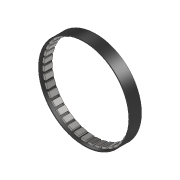
# Autodesk Inventor part: rotor
Saved by Autodesk Inventor 2020 (Build 240168000, 168)
## iProperties
Created: 2020-05-19
Part Number: rotor
Material: Generic
Document SubType Name: Modeling
Designer: Kostic
Density: 1 g/cm^3
Appearance: Glossy - Black
Author: Kostic
Autodesk Inventor part; units mm, degrees
ref_plane "YZ Plane" through (0, 0, 0) normal (1, 0, 0) x (0, 1, 0)
ref_plane "XZ Plane" through (0, 0, 0) normal (0, 1, 0) x (-1, 0, 0)
ref_plane "XY Plane" through (0, 0, 0) normal (0, 0, 1) x (1, 0, 0)
sketch "Sketch1" plane through (0, 0, 0) normal (0, 0, 1) x (1, 0, 0)
  circle A0 centre (0, 0) radius 45.9
  circle A1 centre (0, 0) radius 44.5
  dimension "d0" = 91.8
  dimension "d1" = 89
  constraints: 2 centre point, 2 coincident
  measures "d0" diameter of A0
  measures "d1" diameter of A1
extrude "Extrusion1" add sketch "Sketch1" along normal blind 1
sketch "Sketch2" plane through (0, 0, 1) normal (0, 0, 1) x (1, 0, 0)
  circle A0 centre (0, 0) radius 45.9
  circle A1 centre (0, 0) radius 44.9
  dimension "d4" = 89.8
  dimension "d5" = 91.8
  constraints: 2 centre point, 2 coincident
  measures "d4" diameter of A1
  measures "d5" diameter of A0
extrude "Extrusion2" add sketch "Sketch2" along normal blind 8
sketch "Sketch5" plane through (0, 0, 1) normal (0, 0, 1) x (1, 0, 0)
  line L0 (-2.5, 42.8303) -> (2.5, 42.8303)
  line L1 (2.5, 42.8303) -> (2.5, 44.8303)
  line L2 (2.5, 44.8303) -> (-2.5, 44.8303)
  line L3 (-2.5, 44.8303) -> (-2.5, 42.8303)
  circle A0 centre (0, 0) radius 44.9 projected
  dimension "d8" = 5
  dimension "d9" = 2
  dimension "d10" = 2.5
  constraints: 8 end point, 2 parallel, 1 horizontal, 1 perpendicular, 2 other
  measures "d8" distance of L2.end L1.end
  measures "d9" distance of L1.end L0.end
  measures "d10" distance from line of point (0, 0) L3
extrude "Extrusion3" add sketch "Sketch5" along normal blind 8 contours L3 L2 L1 L0
pattern_circular "Circular Pattern1" count 39 over 360 about axis through (0, 0, 1) along (0, 0, 1) of "Extrusion3"
sketch "Sketch6" plane through (0, 0, 9) normal (0, 0, 1) x (1, 0, 0)
  circle A0 centre (0, 0) radius 45.9
  circle A1 centre (0, 0) radius 44.9
  circle A2 centre (0, 0) radius 45.9 projected
  dimension "d18" = 89.8
  constraints: 2 centre point, 2 coincident, 1 concentric
  measures "d18" diameter of A1
extrude "Extrusion4" add sketch "Sketch6" along normal blind 3
equation "\"d10\" = 0.5 * d8"
body "Solid1"
